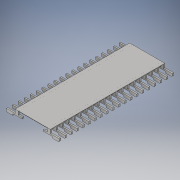
# Autodesk Inventor part: PT-1S39-01(020-01-D-L)
Saved by Autodesk Inventor 2019 (Build 230136000, 136)
## iProperties
Created: 2024-08-20
Part Number: PT-1S39-01(020-01-D-L)
Material: Generic
Catalog Web Link: www.cadenas.de
Description: QTE Series Pin-QTE Series - (0,80 mm) .0315" Q Strip® High Speed Ground Plane Header
Vendor: SAMTEC
Document SubType Name: Modeling
Designer: psAdmin
Manufacturer: SAMTEC
Mass: 0.00896005 g
Surface Area: 2.48699 cm^2
Volume: 0.00896005 cm^3
Density: 1 g/cm^3
Appearance: PSOLRGB-171-171-171
Category: PARTsolutions
Company: SAMTEC
Title: PT-1S39-01(020-01-D-L)
Author: Cadenas PARTsolutions
Comments: QTE Series - (0,80 mm) .0315" Q Strip® High Speed Ground Plane Header
PSOL_IDENT_0: {$CADENAS_DATA/23d-libs/samtec/modelling/qte/parts/qte_pin.prj},208 {VTYP=3D},{NB=PT-1S39-01(020-01-
PSOL_IDENT_1: D-L)},{LINA=PT-1S39-01(020-01-D-L)},{NN=QTE Series Pin},{DATE=14.08.2024 11:26:44},{GEOMDATE=15.07.2
PSOL_IDENT_2: 024 08:40:10},{VERSION=},{LINEID=10},{WBVAR=POS,LS,ROW,PLOPT},{WBNUMERIC=}  {NB=PT-1S39-01(020-01-D-
PSOL_IDENT_3: L)},{LINA=PT-1S39-01(020-01-D-L)},{KT=DUMMY},{PN=T-1S39-01},{SERIES=QTE},{POS=020},{LS=01},{LSALG= '
PSOL_IDENT_4: 01', '-01', '02', '-02', '03', '-03', '04', '-04', '05', '-05'  ,'06','-06', '07', '-07' ,'08','-08'
PSOL_IDENT_5: ,'09','-09','10','-10' },{ROW=D},{ROWALG= 'D','-D - Double' },{PE=0.60650000},{A=0.1680},{H=0.197},{
PSOL_IDENT_6: CH=0.1600},{PLOPT=L},{MAT=samtec_steel_11_07_2024}
NB: PT-1S39-01(020-01-D-L)
NN: QTE Series Pin
NT: QTE Series - (0,80 mm) .0315" Q Strip® High Speed Ground Plane Header
NBSYN: P$PN.($POS.-$LS.-$ROW.-$PLOPT.)
LINA: PT-1S39-01(020-01-D-L)
CATALOG: Samtec
SERIES: QTE
POS: 020
LS: -01
ROW: -D - Double
PLOPT: -L - 10micro" Light Gold in Contact Area, Matte Tin on Tail
SUPPLIER: SAMTEC
ARTICLENO: PT-1S39-01(020-01-D-L)
BOMINFO: PT-1S39-01(020-01-D-L)
CREATOR: CADENAS GmbH
Autodesk Inventor part; units mm, degrees
sketch "Sketch_1" plane through (0, 0, 0) normal (0, 0, 1) x (1, 0, 0)
  arc A0 (-5.6769, -0.0254) -> (-5.5753, -0.127) centre (-5.5753, -0.0254) ccw
  line L0 (-5.5753, -0.127) -> (-4.7879, -0.127)
  line L1 (-4.7879, -0.127) -> (-4.7879, 0.0762)
  line L2 (-4.7879, 0.0762) -> (-3.5433, 0.0762)
  line L3 (-3.5433, 0.0762) -> (-3.5433, 0.254)
  line L4 (-3.5433, 0.254) -> (-4.0894, 0.254)
  line L5 (-4.0894, 0.254) -> (-4.0894, 0.7252)
  line L6 (-4.0894, 0.7252) -> (-0.1524, 0.7252)
  line L7 (-0.1524, 0.7252) -> (-0.1524, 0.254)
  line L8 (-0.1524, 0.254) -> (-0.6985, 0.254)
  line L9 (-0.6985, 0.254) -> (-0.6985, 0.0762)
  line L10 (-0.6985, 0.0762) -> (0.5461, 0.0762)
  line L11 (0.5461, 0.0762) -> (0.5461, -0.127)
  line L12 (0.5461, -0.127) -> (1.3335, -0.127)
  arc A1 (1.3335, -0.127) -> (1.4351, -0.0254) centre (1.3335, -0.0254) ccw
  line L13 (1.4351, -0.0254) -> (1.4351, 0.254)
  line L14 (1.4351, 0.254) -> (0.2413, 0.254)
  line L15 (0.2413, 0.254) -> (0.2413, 3.937)
  arc A2 (0.2413, 3.937) -> (0.1397, 4.0386) centre (0.1397, 3.937) ccw
  line L16 (0.1397, 4.0386) -> (0.0382, 4.0386)
  line L17 (0.0382, 4.0386) -> (-0.1524, 3.7084)
  line L18 (-0.1524, 3.7084) -> (-0.1524, 0.8014)
  line L19 (-0.1524, 0.8014) -> (-4.0894, 0.8014)
  line L20 (-4.0894, 0.8014) -> (-4.0894, 3.7084)
  line L21 (-4.0894, 3.7084) -> (-4.28, 4.0386)
  line L22 (-4.28, 4.0386) -> (-4.3815, 4.0386)
  arc A3 (-4.3815, 4.0386) -> (-4.4831, 3.937) centre (-4.3815, 3.937) ccw
  line L23 (-4.4831, 3.937) -> (-4.4831, 0.254)
  line L24 (-4.4831, 0.254) -> (-5.6769, 0.254)
  line L25 (-5.6769, 0.254) -> (-5.6769, -0.0254)
  constraints: 52 end point, 8 point on circle, 4 centre point
extrude "Extrusion1" add sketch "Sketch_1" against normal blind 15.494
sketch "Sketch_2" plane through (0, 0, 0) normal (1, 0, 0) x (0, 1, 0)
  line L0 (-4.2672, 2.54) -> (-4.2672, -17.78)
  line L1 (-4.2672, -17.78) -> (8.5344, -17.78)
  line L2 (8.5344, -17.78) -> (8.5344, 2.54)
  line L3 (8.5344, 2.54) -> (-4.2672, 2.54)
  line L4 (3.7846, 0) -> (-0.127, 0)
  line L5 (-0.127, 0) -> (-0.127, -0.2032)
  line L6 (-0.127, -0.2032) -> (0.6985, -0.2032)
  line L7 (0.6985, -0.2032) -> (0.6985, -0.8001)
  line L8 (0.6985, -0.8001) -> (-0.127, -0.8001)
  line L9 (-0.127, -0.8001) -> (-0.127, -1.0033)
  line L10 (-0.127, -1.0033) -> (0.6985, -1.0033)
  line L11 (0.6985, -1.0033) -> (0.6985, -1.6002)
  line L12 (0.6985, -1.6002) -> (-0.127, -1.6002)
  line L13 (-0.127, -1.6002) -> (-0.127, -1.8034)
  line L14 (-0.127, -1.8034) -> (0.6985, -1.8034)
  line L15 (0.6985, -1.8034) -> (0.6985, -2.4003)
  line L16 (0.6985, -2.4003) -> (-0.127, -2.4003)
  line L17 (-0.127, -2.4003) -> (-0.127, -2.6035)
  line L18 (-0.127, -2.6035) -> (0.6985, -2.6035)
  line L19 (0.6985, -2.6035) -> (0.6985, -3.2004)
  line L20 (0.6985, -3.2004) -> (-0.127, -3.2004)
  line L21 (-0.127, -3.2004) -> (-0.127, -3.4036)
  line L22 (-0.127, -3.4036) -> (0.6985, -3.4036)
  line L23 (0.6985, -3.4036) -> (0.6985, -4.0005)
  line L24 (0.6985, -4.0005) -> (-0.127, -4.0005)
  line L25 (-0.127, -4.0005) -> (-0.127, -4.2037)
  line L26 (-0.127, -4.2037) -> (0.6985, -4.2037)
  line L27 (0.6985, -4.2037) -> (0.6985, -4.8006)
  line L28 (0.6985, -4.8006) -> (-0.127, -4.8006)
  line L29 (-0.127, -4.8006) -> (-0.127, -5.0038)
  line L30 (-0.127, -5.0038) -> (0.6985, -5.0038)
  line L31 (0.6985, -5.0038) -> (0.6985, -5.6007)
  line L32 (0.6985, -5.6007) -> (-0.127, -5.6007)
  line L33 (-0.127, -5.6007) -> (-0.127, -5.8039)
  line L34 (-0.127, -5.8039) -> (0.6985, -5.8039)
  line L35 (0.6985, -5.8039) -> (0.6985, -6.4008)
  line L36 (0.6985, -6.4008) -> (-0.127, -6.4008)
  line L37 (-0.127, -6.4008) -> (-0.127, -6.604)
  line L38 (-0.127, -6.604) -> (0.6985, -6.604)
  line L39 (0.6985, -6.604) -> (0.6985, -7.2009)
  line L40 (0.6985, -7.2009) -> (-0.127, -7.2009)
  line L41 (-0.127, -7.2009) -> (-0.127, -7.4041)
  line L42 (-0.127, -7.4041) -> (0.6985, -7.4041)
  line L43 (0.6985, -7.4041) -> (0.6985, -8.001)
  line L44 (0.6985, -8.001) -> (-0.127, -8.001)
  line L45 (-0.127, -8.001) -> (-0.127, -8.2042)
  line L46 (-0.127, -8.2042) -> (0.6985, -8.2042)
  line L47 (0.6985, -8.2042) -> (0.6985, -8.8011)
  line L48 (0.6985, -8.8011) -> (-0.127, -8.8011)
  line L49 (-0.127, -8.8011) -> (-0.127, -9.0043)
  line L50 (-0.127, -9.0043) -> (0.6985, -9.0043)
  line L51 (0.6985, -9.0043) -> (0.6985, -9.6012)
  line L52 (0.6985, -9.6012) -> (-0.127, -9.6012)
  line L53 (-0.127, -9.6012) -> (-0.127, -9.8044)
  line L54 (-0.127, -9.8044) -> (0.6985, -9.8044)
  line L55 (0.6985, -9.8044) -> (0.6985, -10.4013)
  line L56 (0.6985, -10.4013) -> (-0.127, -10.4013)
  line L57 (-0.127, -10.4013) -> (-0.127, -10.6045)
  line L58 (-0.127, -10.6045) -> (0.6985, -10.6045)
  line L59 (0.6985, -10.6045) -> (0.6985, -11.2014)
  line L60 (0.6985, -11.2014) -> (-0.127, -11.2014)
  line L61 (-0.127, -11.2014) -> (-0.127, -11.4046)
  line L62 (-0.127, -11.4046) -> (0.6985, -11.4046)
  line L63 (0.6985, -11.4046) -> (0.6985, -12.0015)
  line L64 (0.6985, -12.0015) -> (-0.127, -12.0015)
  line L65 (-0.127, -12.0015) -> (-0.127, -12.2047)
  line L66 (-0.127, -12.2047) -> (0.6985, -12.2047)
  line L67 (0.6985, -12.2047) -> (0.6985, -12.8016)
  line L68 (0.6985, -12.8016) -> (-0.127, -12.8016)
  line L69 (-0.127, -12.8016) -> (-0.127, -13.0048)
  line L70 (-0.127, -13.0048) -> (0.6985, -13.0048)
  line L71 (0.6985, -13.0048) -> (0.6985, -13.6017)
  line L72 (0.6985, -13.6017) -> (-0.127, -13.6017)
  line L73 (-0.127, -13.6017) -> (-0.127, -13.8049)
  line L74 (-0.127, -13.8049) -> (0.6985, -13.8049)
  line L75 (0.6985, -13.8049) -> (0.6985, -14.4018)
  line L76 (0.6985, -14.4018) -> (-0.127, -14.4018)
  line L77 (-0.127, -14.4018) -> (-0.127, -14.605)
  line L78 (-0.127, -14.605) -> (0.6985, -14.605)
  line L79 (0.6985, -14.605) -> (0.6985, -15.2019)
  line L80 (0.6985, -15.2019) -> (-0.127, -15.2019)
  line L81 (-0.127, -15.2019) -> (-0.127, -15.4051)
  line L82 (-0.127, -15.4051) -> (3.7846, -15.4051)
  line L83 (3.7846, -15.4051) -> (4.0386, -15.3543)
  line L84 (4.0386, -15.3543) -> (4.0386, -15.2527)
  line L85 (4.0386, -15.2527) -> (3.7846, -15.2019)
  line L86 (3.7846, -15.2019) -> (0.8255, -15.2019)
  line L87 (0.8255, -15.2019) -> (0.8255, -14.605)
  line L88 (0.8255, -14.605) -> (3.7846, -14.605)
  line L89 (3.7846, -14.605) -> (4.0386, -14.5542)
  line L90 (4.0386, -14.5542) -> (4.0386, -14.4526)
  line L91 (4.0386, -14.4526) -> (3.7846, -14.4018)
  line L92 (3.7846, -14.4018) -> (0.8255, -14.4018)
  line L93 (0.8255, -14.4018) -> (0.8255, -13.8049)
  line L94 (0.8255, -13.8049) -> (3.7846, -13.8049)
  line L95 (3.7846, -13.8049) -> (4.0386, -13.7541)
  line L96 (4.0386, -13.7541) -> (4.0386, -13.6525)
  line L97 (4.0386, -13.6525) -> (3.7846, -13.6017)
  line L98 (3.7846, -13.6017) -> (0.8255, -13.6017)
  line L99 (0.8255, -13.6017) -> (0.8255, -13.0048)
  line L100 (0.8255, -13.0048) -> (3.7846, -13.0048)
  line L101 (3.7846, -13.0048) -> (4.0386, -12.954)
  line L102 (4.0386, -12.954) -> (4.0386, -12.8524)
  line L103 (4.0386, -12.8524) -> (3.7846, -12.8016)
  line L104 (3.7846, -12.8016) -> (0.8255, -12.8016)
  line L105 (0.8255, -12.8016) -> (0.8255, -12.2047)
  line L106 (0.8255, -12.2047) -> (3.7846, -12.2047)
  line L107 (3.7846, -12.2047) -> (4.0386, -12.1539)
  line L108 (4.0386, -12.1539) -> (4.0386, -12.0523)
  line L109 (4.0386, -12.0523) -> (3.7846, -12.0015)
  line L110 (3.7846, -12.0015) -> (0.8255, -12.0015)
  line L111 (0.8255, -12.0015) -> (0.8255, -11.4046)
  line L112 (0.8255, -11.4046) -> (3.7846, -11.4046)
  line L113 (3.7846, -11.4046) -> (4.0386, -11.3538)
  line L114 (4.0386, -11.3538) -> (4.0386, -11.2522)
  line L115 (4.0386, -11.2522) -> (3.7846, -11.2014)
  line L116 (3.7846, -11.2014) -> (0.8255, -11.2014)
  line L117 (0.8255, -11.2014) -> (0.8255, -10.6045)
  line L118 (0.8255, -10.6045) -> (3.7846, -10.6045)
  line L119 (3.7846, -10.6045) -> (4.0386, -10.5537)
  line L120 (4.0386, -10.5537) -> (4.0386, -10.4521)
  line L121 (4.0386, -10.4521) -> (3.7846, -10.4013)
  line L122 (3.7846, -10.4013) -> (0.8255, -10.4013)
  line L123 (0.8255, -10.4013) -> (0.8255, -9.8044)
  line L124 (0.8255, -9.8044) -> (3.7846, -9.8044)
  line L125 (3.7846, -9.8044) -> (4.0386, -9.7536)
  line L126 (4.0386, -9.7536) -> (4.0386, -9.652)
  line L127 (4.0386, -9.652) -> (3.7846, -9.6012)
  line L128 (3.7846, -9.6012) -> (0.8255, -9.6012)
  line L129 (0.8255, -9.6012) -> (0.8255, -9.0043)
  line L130 (0.8255, -9.0043) -> (3.7846, -9.0043)
  line L131 (3.7846, -9.0043) -> (4.0386, -8.9535)
  line L132 (4.0386, -8.9535) -> (4.0386, -8.8519)
  line L133 (4.0386, -8.8519) -> (3.7846, -8.8011)
  line L134 (3.7846, -8.8011) -> (0.8255, -8.8011)
  line L135 (0.8255, -8.8011) -> (0.8255, -8.2042)
  line L136 (0.8255, -8.2042) -> (3.7846, -8.2042)
  line L137 (3.7846, -8.2042) -> (4.0386, -8.1534)
  line L138 (4.0386, -8.1534) -> (4.0386, -8.0518)
  line L139 (4.0386, -8.0518) -> (3.7846, -8.001)
  line L140 (3.7846, -8.001) -> (0.8255, -8.001)
  line L141 (0.8255, -8.001) -> (0.8255, -7.4041)
  line L142 (0.8255, -7.4041) -> (3.7846, -7.4041)
  line L143 (3.7846, -7.4041) -> (4.0386, -7.3533)
  line L144 (4.0386, -7.3533) -> (4.0386, -7.2517)
  line L145 (4.0386, -7.2517) -> (3.7846, -7.2009)
  line L146 (3.7846, -7.2009) -> (0.8255, -7.2009)
  line L147 (0.8255, -7.2009) -> (0.8255, -6.604)
  line L148 (0.8255, -6.604) -> (3.7846, -6.604)
  line L149 (3.7846, -6.604) -> (4.0386, -6.5532)
  line L150 (4.0386, -6.5532) -> (4.0386, -6.4516)
  line L151 (4.0386, -6.4516) -> (3.7846, -6.4008)
  line L152 (3.7846, -6.4008) -> (0.8255, -6.4008)
  line L153 (0.8255, -6.4008) -> (0.8255, -5.8039)
  line L154 (0.8255, -5.8039) -> (3.7846, -5.8039)
  line L155 (3.7846, -5.8039) -> (4.0386, -5.7531)
  line L156 (4.0386, -5.7531) -> (4.0386, -5.6515)
  line L157 (4.0386, -5.6515) -> (3.7846, -5.6007)
  line L158 (3.7846, -5.6007) -> (0.8255, -5.6007)
  line L159 (0.8255, -5.6007) -> (0.8255, -5.0038)
  line L160 (0.8255, -5.0038) -> (3.7846, -5.0038)
  line L161 (3.7846, -5.0038) -> (4.0386, -4.953)
  line L162 (4.0386, -4.953) -> (4.0386, -4.8514)
  line L163 (4.0386, -4.8514) -> (3.7846, -4.8006)
  line L164 (3.7846, -4.8006) -> (0.8255, -4.8006)
  line L165 (0.8255, -4.8006) -> (0.8255, -4.2037)
  line L166 (0.8255, -4.2037) -> (3.7846, -4.2037)
  line L167 (3.7846, -4.2037) -> (4.0386, -4.1529)
  line L168 (4.0386, -4.1529) -> (4.0386, -4.0513)
  line L169 (4.0386, -4.0513) -> (3.7846, -4.0005)
  line L170 (3.7846, -4.0005) -> (0.8255, -4.0005)
  line L171 (0.8255, -4.0005) -> (0.8255, -3.4036)
  line L172 (0.8255, -3.4036) -> (3.7846, -3.4036)
  line L173 (3.7846, -3.4036) -> (4.0386, -3.3528)
  line L174 (4.0386, -3.3528) -> (4.0386, -3.2512)
  line L175 (4.0386, -3.2512) -> (3.7846, -3.2004)
  line L176 (3.7846, -3.2004) -> (0.8255, -3.2004)
  line L177 (0.8255, -3.2004) -> (0.8255, -2.6035)
  line L178 (0.8255, -2.6035) -> (3.7846, -2.6035)
  line L179 (3.7846, -2.6035) -> (4.0386, -2.5527)
  line L180 (4.0386, -2.5527) -> (4.0386, -2.4511)
  line L181 (4.0386, -2.4511) -> (3.7846, -2.4003)
  line L182 (3.7846, -2.4003) -> (0.8255, -2.4003)
  line L183 (0.8255, -2.4003) -> (0.8255, -1.8034)
  line L184 (0.8255, -1.8034) -> (3.7846, -1.8034)
  line L185 (3.7846, -1.8034) -> (4.0386, -1.7526)
  line L186 (4.0386, -1.7526) -> (4.0386, -1.651)
  line L187 (4.0386, -1.651) -> (3.7846, -1.6002)
  line L188 (3.7846, -1.6002) -> (0.8255, -1.6002)
  line L189 (0.8255, -1.6002) -> (0.8255, -1.0033)
  line L190 (0.8255, -1.0033) -> (3.7846, -1.0033)
  line L191 (3.7846, -1.0033) -> (4.0386, -0.9525)
  line L192 (4.0386, -0.9525) -> (4.0386, -0.8509)
  line L193 (4.0386, -0.8509) -> (3.7846, -0.8001)
  line L194 (3.7846, -0.8001) -> (0.8255, -0.8001)
  line L195 (0.8255, -0.8001) -> (0.8255, -0.2032)
  line L196 (0.8255, -0.2032) -> (3.7846, -0.2032)
  line L197 (3.7846, -0.2032) -> (4.0386, -0.1524)
  line L198 (4.0386, -0.1524) -> (4.0386, -0.0508)
  line L199 (4.0386, -0.0508) -> (3.7846, 0)
  constraints: 400 end point
extrude "Extrusion2" cut sketch "Sketch_2" along normal mid plane 50.8
sketch "Sketch_5" plane through (0, 0, 0) normal (0, 0, 1) x (1, 0, 0)
  line L0 (-508, 1016.762) -> (-508, 0.762)
  line L1 (-508, 0.762) -> (508, 0.762)
  line L2 (508, 0.762) -> (508, 1016.762)
  line L3 (508, 1016.762) -> (-508, 1016.762)
  constraints: 8 end point
extrude "Extrusion3" cut sketch "Sketch_5" along normal mid plane 2540
ref_plane "p1_to_p2_XY" through (0, 0, 0) normal (0, 1, 0) x (1, 0, 0)
ref_plane "p1_to_p2_YZ" through (0, 0, 0) normal (1, 0, 0) x (0, 0, -1)
ref_plane "p1_to_p2_ZX" through (0, 0, 0) normal (0, 0, -1) x (0, 1, 0)
ref_plane "pin_XY" through (1.4351, 0.254, 0.0571) normal (0, 1, 0) x (1, 0, 0)
ref_plane "pin_YZ" through (1.4351, 0.254, 0.0571) normal (1, 0, 0) x (0, 0, -1)
ref_plane "pin_ZX" through (1.4351, 0.254, 0.0571) normal (0, 0, -1) x (0, 1, 0)
body "Solid1"
